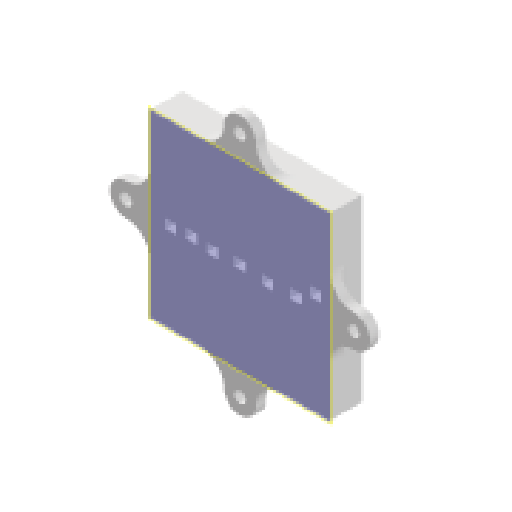
# Autodesk Inventor part: frame
Saved by Autodesk Inventor 2023 (Build 270158030, 158C)
## iProperties
Created: 2022-08-19
Part Number: frame
Material: Generic
Document SubType Name: Modeling
Designer: James
Density: 1 g/cm^3
Appearance: Default
Author: James
Autodesk Inventor part; units mm, degrees
ref_plane "YZ Plane" through (0, 0, 0) normal (1, 0, 0) x (0, 1, 0)
ref_plane "XZ Plane" through (0, 0, 0) normal (0, 1, 0) x (-1, 0, 0)
ref_plane "XY Plane" through (0, 0, 0) normal (0, 0, 1) x (1, 0, 0)
sketch "Sketch1" plane through (0, 0, 0) normal (0, 0, 1) x (1, 0, 0)
  circle A0 centre (23.5812, 3.9705) radius 1.4165 construction
  circle A1 centre (17.25, 0) radius 1.4165 construction
  circle A2 centre (8.575, 0) radius 1.4165 construction
  circle A3 centre (0, 0) radius 1.4165 construction
  circle A4 centre (-8.4745, 0) radius 1.4165 construction
  circle A5 centre (-15.0058, 0) radius 1.4165 construction
  circle A6 centre (-21.437, 0) radius 1.4165 construction
  line L0 (25.625, 25.625) -> (-25.6245, 25.625) construction
  line L1 (-25.6245, 25.625) -> (-25.6245, -25.625) construction
  line L2 (-25.6245, -25.625) -> (25.625, -25.625) construction
  line L3 (25.625, -25.625) -> (25.625, 25.625) construction
  line L4 (21.8312, 5.4035) -> (25.3312, 5.4035)
  line L5 (25.3312, 5.4035) -> (25.3312, 2.5375)
  line L6 (25.3312, 2.5375) -> (21.8312, 2.5375)
  line L7 (21.8312, 2.5375) -> (21.8312, 5.4035)
  line L8 (21.8312, 5.4035) -> (25.3312, 2.5375) construction
  line L9 (25.3312, 5.4035) -> (21.8312, 2.5375) construction
  line L10 (15.5, 1.75) -> (19, 1.75)
  line L11 (19, 1.75) -> (19, -1.116)
  line L12 (15.5, -1.116) -> (15.5, 1.75)
  line L13 (6.825, 1.116) -> (10.325, 1.116)
  line L14 (10.325, 1.116) -> (10.325, -1.75)
  line L15 (10.325, -1.75) -> (6.825, -1.75)
  line L16 (6.825, -1.75) -> (6.825, 1.116)
  line L17 (-1.75, 1.75) -> (1.75, 1.75)
  line L18 (1.75, 1.75) -> (1.75, -1.116)
  line L19 (-1.75, -1.116) -> (-1.75, 1.75)
  line L20 (-10.2245, 1.116) -> (-6.7245, 1.116)
  line L21 (-6.7245, 1.116) -> (-6.7245, -1.75)
  line L22 (-6.7245, -1.75) -> (-10.2245, -1.75)
  line L23 (-10.2245, -1.75) -> (-10.2245, 1.116)
  line L24 (-16.7558, 1.75) -> (-13.2558, 1.75)
  line L25 (-13.2558, 1.75) -> (-13.2558, -1.116)
  line L26 (-16.7558, -1.116) -> (-16.7558, 1.75)
  line L27 (-23.187, 1.116) -> (-19.687, 1.116)
  line L28 (-19.687, 1.116) -> (-19.687, -1.75)
  line L29 (-19.687, -1.75) -> (-23.187, -1.75)
  line L30 (-23.187, -1.75) -> (-23.187, 1.116)
  line L31 (25.825, 25.825) -> (-25.8245, 25.825)
  line L32 (-25.8245, 25.825) -> (-25.8245, -25.825)
  line L33 (-25.8245, -25.825) -> (25.825, -25.825)
  line L34 (25.825, -25.825) -> (25.825, 25.825)
  line L35 (27.825, 27.825) -> (-27.8245, 27.825)
  line L36 (-27.8245, 27.825) -> (-27.8245, -27.825)
  line L37 (-27.8245, -27.825) -> (27.825, -27.825)
  line L38 (27.825, -27.825) -> (27.825, 27.825)
  line L39 (-16.7558, -1.116) -> (-13.2558, -1.116)
  line L40 (-1.75, -1.116) -> (1.75, -1.116)
  line L41 (15.5, -1.116) -> (19, -1.116)
  point P0 (0, 0)
  point P1 (-16.6189, -1.116)
  dimension "d0" = 3.5
  dimension "d1" = 2.866
  dimension "d4" = 3.5
  dimension "d5" = 2.866
  dimension "d8" = 3.5
  dimension "d9" = 2.866
  dimension "d12" = 3.5
  dimension "d13" = 2.866
  dimension "d14" = 0.2
  dimension "d15" = 2
  constraints: 84 end point, 11 parallel, 8 perpendicular, 7 centre point, 7 horizontal, 4 point on line, 2 midpoint, 6 other
  measures "d0" distance of L5.end L6.end
  measures "d1" distance of L4.end L5.end
  measures "d4" distance of L14.end L16.start
  measures "d5" distance of L13.end L14.end
  measures "d8" distance of L21.end L23.start
  measures "d9" distance of L20.end L21.end
  measures "d12" distance of L28.end L30.start
  measures "d13" distance of L27.end L28.end
  measures "d14" distance between parallel lines of L3 L34
  measures "d15" distance between parallel lines of L34 L38
extrude "Extrusion1" add sketch "Sketch1" along normal blind 10 contours L34 L33 L32 L31 | L38 L37 L36 L35
sketch "Sketch2" plane through (0, 0, 0) normal (0, 0, -1) x (-1, 0, 0)
  line L0 (27.8245, 27.825) -> (27.8245, -27.825) projected
  line L1 (-27.825, 27.825) -> (27.8245, 27.825) projected
  line L2 (-27.825, -27.825) -> (-27.825, 27.825) projected
  line L3 (27.8245, -27.825) -> (-27.825, -27.825) projected
  line L4 (23.187, -1.75) -> (23.187, 1.116) projected
  line L5 (19.687, -1.75) -> (23.187, -1.75) projected
  line L6 (19.687, 1.116) -> (19.687, -1.75) projected
  line L7 (23.187, 1.116) -> (19.687, 1.116) projected
  line L8 (10.2245, -1.75) -> (10.2245, 1.116) projected
  line L9 (6.7245, -1.75) -> (10.2245, -1.75) projected
  line L10 (6.7245, 1.116) -> (6.7245, -1.75) projected
  line L11 (10.2245, 1.116) -> (6.7245, 1.116) projected
  line L12 (-6.825, -1.75) -> (-6.825, 1.116) projected
  line L13 (-10.325, -1.75) -> (-6.825, -1.75) projected
  line L14 (-10.325, 1.116) -> (-10.325, -1.75) projected
  line L15 (-6.825, 1.116) -> (-10.325, 1.116) projected
  line L16 (-21.8312, 5.4035) -> (-25.3312, 5.4035) projected
  line L17 (-21.8312, 2.5375) -> (-21.8312, 5.4035) projected
  line L18 (-25.3312, 2.5375) -> (-21.8312, 2.5375) projected
  line L19 (-25.3312, 5.4035) -> (-25.3312, 2.5375) projected
  line L20 (25.8245, -25.825) -> (25.8245, 25.825)
  line L21 (25.8245, 25.825) -> (-25.825, 25.825)
  line L22 (-25.825, 25.825) -> (-25.825, -25.825)
  line L23 (-25.825, -25.825) -> (25.8245, -25.825)
  point P0 (0, 0)
  dimension "d18" = 2
  constraints: 8 end point, 3 other
  measures "d18" distance between parallel lines of L0 L20
extrude "Extrusion2" [suppressed]
ref_plane "Work Plane1" through (0, 0, 10) normal (0, 0, -1) x (-1, 0, 0)
sketch "Sketch3" plane through (0, 0, 10) normal (0, 0, -1) x (-1, 0, 0)
  circle A0 centre (35.325, 0) radius 1.75
  circle A1 centre (-0.0002, -35.325) radius 1.75
  circle A2 centre (-35.325, 0) radius 1.75
  circle A3 centre (-0.0002, 35.325) radius 1.75
  line L0 (7.4998, 35.325) -> (7.4998, 35.325)
  line L1 (-7.5003, 35.325) -> (-7.5003, 35.325)
  arc A4 (4.9998, 35.325) -> (-5.0002, 35.325) centre (-0.0002, 35.325) ccw
  arc A5 (-35.325, 5) -> (-35.325, -5) centre (-35.325, 0) ccw
  arc A6 (35.325, -5) -> (35.325, 5) centre (35.325, 0) ccw
  arc A7 (-5.0002, -35.325) -> (4.9998, -35.325) centre (-0.0002, -35.325) ccw
  line L2 (27.8245, 27.825) -> (-27.825, 27.825) projected
  line L3 (27.8245, -27.825) -> (-27.825, -27.825) projected
  line L4 (-35.325, 5) -> (-35.325, 5)
  line L5 (-5.0002, 35.325) -> (-5.0002, 35.325)
  line L6 (4.9998, 35.325) -> (4.9998, 35.325)
  line L7 (35.325, 5) -> (35.3245, 5)
  line L8 (27.8245, -27.825) -> (27.8245, 27.825) projected
  line L9 (35.325, -5) -> (35.3245, -5)
  line L10 (4.9998, -35.325) -> (4.9998, -35.325)
  line L11 (-5.0002, -35.325) -> (-5.0002, -35.325)
  line L12 (-35.325, -5) -> (-35.325, -5)
  line L13 (-27.825, -27.825) -> (-27.825, -12.5)
  line L14 (-27.825, 12.5) -> (-27.825, 27.825)
  line L15 (27.8245, -27.825) -> (12.4998, -27.825)
  line L16 (-12.5002, -27.825) -> (-27.825, -27.825)
  line L17 (27.8245, 27.825) -> (27.8245, 12.5)
  line L18 (27.8245, -12.5) -> (27.8245, -27.825)
  line L19 (-27.825, 27.825) -> (-12.5002, 27.825)
  line L20 (12.4998, 27.825) -> (27.8245, 27.825)
  arc A8 (-35.325, 5) -> (-27.825, 12.5) centre (-35.325, 12.5) ccw
  arc A9 (-27.825, -12.5) -> (-35.325, -5) centre (-35.325, -12.5) ccw
  arc A10 (-5.0002, -35.325) -> (-12.5002, -27.825) centre (-12.5002, -35.325) ccw
  arc A11 (12.4998, -27.825) -> (4.9998, -35.325) centre (12.4998, -35.325) ccw
  arc A12 (35.3245, -5) -> (27.8245, -12.5) centre (35.3245, -12.5) ccw
  arc A13 (27.8245, 12.5) -> (35.3245, 5) centre (35.3245, 12.5) ccw
  arc A14 (4.9998, 35.325) -> (12.4998, 27.825) centre (12.4998, 35.325) ccw
  arc A15 (-12.5002, 27.825) -> (-5.0002, 35.325) centre (-12.5002, 35.325) ccw
  line L21 (-27.825, -12.5) -> (-27.825, 12.5)
  line L22 (-25.825, -25.825) -> (-25.825, 25.825) projected
  point P0 (27.8245, 5)
  point P1 (27.8245, -5)
  point P2 (-5.0002, -35.325)
  point P3 (4.9998, -35.325)
  point P4 (-5.0002, 35.325)
  dimension "d25" = 10
  dimension "d26" = 10
  dimension "d27" = 7.5
  constraints: 38 end point, 24 point on circle, 21 tangent, 16 centre point, 12 perpendicular, 10 parallel, 7 equal radius, 6 coincident, 6 point on line, 4 horizontal
  measures "d25" diameter of A4
  measures "d26" diameter of A5
  measures "d27" radius of A8
extrude "Extrusion3" add sketch "Sketch3" along normal blind 3 contours A14 L2 A15 A4 | A13 A6 A12 L8 | L21 A9 A5 A8 | A11 A7 A10 L3
fillet "Fillet1" radius 2 4 edges at (-27.8245, 0, 7) (0.0002, 27.825, 7) (27.825, 0, 7) (0.0002, -27.825, 7)
sketch "Sketch4" plane through (0, 0, 0) normal (0, 0, -1) x (-1, 0, 0)
  line L0 (27.8245, 27.825) -> (27.8245, -27.825) construction
  line L1 (-27.825, 27.825) -> (27.8245, 27.825) construction
  line L2 (-27.825, -27.825) -> (-27.825, 27.825) construction
  line L3 (27.8245, -27.825) -> (-27.825, -27.825) construction
  line L4 (-21.8312, 5.4035) -> (-25.3312, 5.4035) construction
  line L5 (-21.8312, 2.5375) -> (-21.8312, 5.4035) construction
  line L6 (-25.3312, 2.5375) -> (-21.8312, 2.5375) construction
  line L7 (-25.3312, 5.4035) -> (-25.3312, 2.5375) construction
  line L8 (-15.5, -1.116) -> (-15.5, 1.75) construction
  line L9 (-19, -1.116) -> (-15.5, -1.116) construction
  line L10 (-19, 1.75) -> (-19, -1.116) construction
  line L11 (-15.5, 1.75) -> (-19, 1.75) construction
  line L12 (-6.825, -1.75) -> (-6.825, 1.116) construction
  line L13 (-10.325, -1.75) -> (-6.825, -1.75) construction
  line L14 (-10.325, 1.116) -> (-10.325, -1.75) construction
  line L15 (-6.825, 1.116) -> (-10.325, 1.116) construction
  line L16 (1.75, -1.116) -> (1.75, 1.75) construction
  line L17 (-1.75, -1.116) -> (1.75, -1.116) construction
  line L18 (-1.75, 1.75) -> (-1.75, -1.116) construction
  line L19 (1.75, 1.75) -> (-1.75, 1.75) construction
  line L20 (10.2245, -1.75) -> (10.2245, 1.116) construction
  line L21 (6.7245, -1.75) -> (10.2245, -1.75) construction
  line L22 (6.7245, 1.116) -> (6.7245, -1.75) construction
  line L23 (10.2245, 1.116) -> (6.7245, 1.116) construction
  line L24 (16.7558, -1.116) -> (16.7558, 1.75) construction
  line L25 (13.2558, -1.116) -> (16.7558, -1.116) construction
  line L26 (13.2558, 1.75) -> (13.2558, -1.116) construction
  line L27 (16.7558, 1.75) -> (13.2558, 1.75) construction
  line L28 (23.187, -1.75) -> (23.187, 1.116) construction
  line L29 (19.687, -1.75) -> (23.187, -1.75) construction
  line L30 (19.687, 1.116) -> (19.687, -1.75) construction
  line L31 (23.187, 1.116) -> (19.687, 1.116) construction
  line L32 (26.8245, -26.825) -> (26.8245, 26.825)
  line L33 (26.8245, 26.825) -> (-26.825, 26.825)
  line L34 (-26.825, 26.825) -> (-26.825, -26.825)
  line L35 (-26.825, -26.825) -> (26.8245, -26.825)
  line L36 (24.187, -2.75) -> (24.187, 2.116)
  line L37 (18.687, 2.116) -> (18.687, -2.75)
  line L38 (17.7558, -2.116) -> (17.7558, 2.75)
  line L39 (12.2558, 2.75) -> (12.2558, -2.116)
  line L40 (11.2245, -2.75) -> (11.2245, 2.116)
  line L41 (5.7245, 2.116) -> (5.7245, -2.75)
  line L42 (2.75, -2.116) -> (2.75, 2.75)
  line L43 (-2.75, 2.75) -> (-2.75, -2.116)
  line L44 (-5.825, -2.75) -> (-5.825, 2.116)
  line L45 (-11.325, 2.116) -> (-11.325, -2.75)
  line L46 (-14.5, 2.75) -> (-14.5, -2.116)
  line L47 (-20, -2.116) -> (-20, 2.75)
  line L48 (-20.8312, 1.5375) -> (-20.8312, 6.4035)
  line L49 (-26.3312, 6.4035) -> (-26.3312, 1.5375)
  line L50 (-23.5812, 26.825) -> (-23.5812, -26.825) construction
  line L51 (-17.25, 26.825) -> (-17.25, -26.825) construction
  line L52 (-0.0002, 26.825) -> (-0.0003, -26.825) construction
  line L53 (8.4745, -26.825) -> (8.4745, 26.825) construction
  line L54 (15.0058, 26.825) -> (15.0057, -26.825) construction
  line L55 (21.437, -26.825) -> (21.437, 26.825) construction
  line L56 (-22.5812, 26.825) -> (-22.5812, 6.4035)
  line L57 (-22.5812, 1.5375) -> (-22.5812, -26.825)
  line L58 (-24.5812, 26.825) -> (-24.5812, 6.4035)
  line L59 (-24.5812, 1.5375) -> (-24.5812, -26.825)
  line L60 (-26.3312, 1.5375) -> (-24.5812, 1.5375)
  line L61 (-22.5812, 1.5375) -> (-20.8312, 1.5375)
  line L62 (-20.8312, 6.4035) -> (-22.5812, 6.4035)
  line L63 (-24.5812, 6.4035) -> (-26.3312, 6.4035)
  line L64 (-20, 2.75) -> (-18.25, 2.75)
  line L65 (-16.25, 2.75) -> (-14.5, 2.75)
  line L66 (-16.25, 26.825) -> (-16.25, 2.75)
  line L67 (-16.25, -2.116) -> (-16.25, -26.825)
  line L68 (-18.25, 26.825) -> (-18.25, 2.75)
  line L69 (-18.25, -2.116) -> (-18.25, -26.825)
  line L70 (-14.5, -2.116) -> (-16.25, -2.116)
  line L71 (-18.25, -2.116) -> (-20, -2.116)
  line L72 (-11.325, -2.75) -> (-9.575, -2.75)
  line L73 (-7.575, -2.75) -> (-5.825, -2.75)
  line L74 (-5.825, 2.116) -> (-7.575, 2.116)
  line L75 (-9.575, 2.116) -> (-11.325, 2.116)
  line L76 (2.75, 2.75) -> (0.9998, 2.75)
  line L77 (-1.0002, 2.75) -> (-2.75, 2.75)
  line L78 (0.9998, 26.825) -> (0.9998, 2.75)
  line L79 (0.9998, -2.116) -> (0.9998, -26.825)
  line L80 (-2.75, -2.116) -> (-1.0002, -2.116)
  line L81 (0.9998, -2.116) -> (2.75, -2.116)
  line L82 (-1.0002, 26.825) -> (-1.0002, 2.75)
  line L83 (-1.0002, -2.116) -> (-1.0002, -26.825)
  line L84 (11.2245, 2.116) -> (9.4745, 2.116)
  line L85 (7.4745, 2.116) -> (5.7245, 2.116)
  line L86 (9.4745, -26.825) -> (9.4745, -2.75)
  line L87 (9.4745, 2.116) -> (9.4745, 26.825)
  line L88 (5.7245, -2.75) -> (7.4745, -2.75)
  line L89 (9.4745, -2.75) -> (11.2245, -2.75)
  line L90 (7.4745, -26.825) -> (7.4745, -2.75)
  line L91 (7.4745, 2.116) -> (7.4745, 26.825)
  line L92 (14.0058, 26.825) -> (14.0058, 2.75)
  line L93 (16.0058, 26.825) -> (16.0058, 2.75)
  line L94 (16.0058, -2.116) -> (16.0057, -26.825)
  line L95 (14.0058, -2.116) -> (14.0057, -26.825)
  line L96 (20.437, 2.116) -> (20.437, 26.825)
  line L97 (22.437, -26.825) -> (22.437, -2.75)
  line L98 (22.437, 2.116) -> (22.437, 26.825)
  line L99 (24.187, 2.116) -> (22.437, 2.116)
  line L100 (20.437, 2.116) -> (18.687, 2.116)
  line L101 (17.7558, 2.75) -> (16.0058, 2.75)
  line L102 (14.0058, 2.75) -> (12.2558, 2.75)
  line L103 (12.2558, -2.116) -> (14.0058, -2.116)
  line L104 (16.0058, -2.116) -> (17.7558, -2.116)
  line L105 (20.437, -26.825) -> (20.437, -2.75)
  line L106 (18.687, -2.75) -> (20.437, -2.75)
  line L107 (22.437, -2.75) -> (24.187, -2.75)
  line L108 (-8.575, 26.825) -> (-8.575, -26.825) construction
  line L109 (-7.575, 26.825) -> (-7.575, 2.116)
  line L110 (-7.575, -2.75) -> (-7.575, -26.825)
  line L111 (-9.575, 26.825) -> (-9.575, 2.116)
  line L112 (-9.575, -2.75) -> (-9.575, -26.825)
  point P0 (0, 0)
  dimension "d4" = 3.5
  dimension "d5" = 2.866
  constraints: 158 end point, 28 parallel, 5 vertical, 1 perpendicular, 23 other
extrude "Extrusion4" [suppressed]
body "Solid1"
